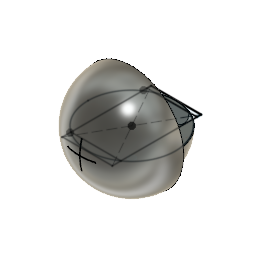
led-juggling-ball (Autodesk Fusion 360 design; units mm, degrees)
Autodesk Fusion 360 part; units mm, degrees
sketch "Sketch1" plane through (0, 0, 0) normal (0, 0, 1) x (1, 0, 0)
  circle A0 centre (0, 0) radius 37.5
  line L0 (-37.5, 0) -> (37.5, 0)
  circle A1 centre (0, 0) radius 33.25
  line L1 (-32.8653, 0.0244) -> (-33.25, 0)
  line L2 (0, 37.5) -> (0, 0)
  line L3 (0, 0) -> (0, -37.5)
  dimension "d1" = 75
  dimension "d2" = 66.5
  constraint coincident A0.centre A1.centre
  constraint coincident A0 L0.start
  constraint coincident A0 L0.end
  constraint horizontal L0
  constraint concentric A0 A1
  constraint coincident A1 L1.end
  constraint coincident L0 L1.end
  constraint coincident A0 L2.start
  constraint coincident A0 L3.end
  constraint perpendicular L0 L3
  measures "d1" diameter of A0
  measures "d2" diameter of A1
revolve "Revolve3" add sketch "Sketch1" angle 360 about axis through (0, 0, 0) along (0, -1, 0) contours A0 L0 A1 L3 picked at (-3.3563, -35.8433) makes body 1
revolve "Revolve2" add sketch "Sketch1" angle 360 about axis through (0, 37.5, 0) along (0, -1, 0) separate body contours A0 L0 A1 L2 picked at (-1.7789, 35.9561) makes body 2
sketch "Sketch2" plane through (0, 0, 0) normal (0, 1, 0) x (1, 0, 0)
  circle A0 centre (0, 0) radius 10
  dimension "d7" = 20
  constraint coincident A0.centre origin
  measures "d7" diameter of A0
extrude "Extrude1" cut sketch "Sketch2" against normal blind 60 bodies 1
sketch "Sketch3" plane through (0, 0, 0) normal (0, 0, 1) x (1, 0, 0)
  spline S0 degree 5 poles (0, -35) (0.4009, -35.0057) (1.2027, -35.0023) (2.4054, -34.9527) (4.0091, -34.8067) (6.012, -34.5127) (7.6108, -34.1894) (8.8068, -33.8887) (9.6025, -33.6595) (10, -33.5378) knots 0 0 0 0 0 0 0.2 0.4 0.6 0.8 1 1 1 1 1 1
  line L0 (-1.0163, -34.9855) -> (1.0163, -35.0145)
  line L1 (8.9918, -33.8467) -> (11.0081, -33.2288)
  line L2 (0, -35) -> (0, -31.5)
  line L3 (10, -33.5378) -> (10, -29.5378)
  line L4 (10, -29.5378) -> (11.8793, -28.8537)
  line L5 (11.8793, -28.8537) -> (11.8793, -28.4537)
  spline S1 degree 5 poles (11.8793, -28.4537) (11.8793, -28.4528) (11.7956, -28.4591) (11.4191, -28.4933) (10.6251, -28.5552) (9.9506, -28.5569) (9.9154, -28.5174) (9.5374, -28.7608) (8.5649, -29.3019) (6.9381, -30.0477) (4.8211, -30.8112) (2.912, -31.2735) (1.4544, -31.4588) (0.4845, -31.5) (0, -31.5) knots 0 0 0 0 0 0 0.1 0.2 0.3 0.4 0.5 0.6 0.7 0.8 0.9 1 1 1 1 1 1
  line L6 (10.242, -28.5357) -> (9.7191, -28.5641)
  line L7 (11.8793, -28.4607) -> (11.8793, -28.4468)
  line L8 (1.9201, -31.5) -> (-1.9201, -31.5)
  point P0 (9.9806, -28.5499)
  dimension "d10" = 4
  dimension "d11" = 110
  dimension "d12" = 2
  dimension "d13" = 0.4
  dimension "d61" = 3.5
  constraint midpoint S0.start L0
  constraint midpoint S0.end L1
  constraint vertical L3
  constraint vertical L5
  constraint midpoint P0 L6
  constraint midpoint L5.end L7
  constraint coincident L6 L7.end
  constraint midpoint L2.end L8
  constraint coincident L5 L7.start
  measures "d10" distance of S0.end L3.end
  measures "d11" angle of L3 L4
  measures "d12" distance of L3.end L4.end
  measures "d13" distance of L4.end L5.end
  measures "d61" distance of S0.start L2.end
sketch "Sketch4" plane through (0, 0, 0) normal (0, 0, 1) x (1, 0, 0)
  line L0 (10, -33.5) -> (10, -30.5)
  spline S0 degree 5 poles (0, -35) (0.3549, -35) (1.0653, -34.9917) (2.133, -34.9543) (3.5701, -34.8539) (5.4548, -34.6187) (7.113, -34.2978) (8.4939, -33.948) (9.486, -33.6587) (10, -33.5) knots 0 0 0 0 0 0 0.2 0.4 0.6 0.8 1 1 1 1 1 1
  line L1 (8.6967, -33.9024) -> (11.3033, -33.0976)
  line L2 (-0.9, -35) -> (0.9, -35)
  line L3 (10, -30.5) -> (8, -30.5)
  line L4 (0, -35) -> (0, -33)
  spline S1 degree 5 poles (0, -33) (0.7014, -32.9425) (1.9674, -32.8352) (3.4564, -32.6972) (4.7558, -32.5362) (5.7676, -32.2435) (6.495, -31.7925) (7.1733, -31.2433) (7.7103, -30.7663) (8, -30.5) knots 0 0 0 0 0 0 0.2 0.4 0.6 0.8 1 1 1 1 1 1
  line L5 (-1.7671, -33.1448) -> (1.7671, -32.8552)
  line L6 (7.2949, -31.1481) -> (8.7051, -29.8519)
  dimension "d15" = 3
  dimension "d22" = 2
  constraint vertical L0
  constraint midpoint L0.start L1
  constraint midpoint S0.start L2
  constraint perpendicular L0 L3
  constraint vertical L4
  constraint midpoint L4.end L5
  constraint midpoint L3.end L6
  measures "d15" distance of L0.start L0.end
  measures "d22" distance of L0.end L3.end
sketch "Sketch6" plane through (0, 0, 0) normal (0, 1, 0) x (1, 0, 0)
  line L0 (-32, 0) -> (0, 0)
  line L1 (0, 0) -> (0, 32)
  circle A0 centre (0, 0) radius 32
  dimension "d103" = 64
  constraint coincident L0.end L1.start
  constraint horizontal L0
  constraint perpendicular L0 L1
  constraint coincident L1.end A0
  measures "d103" diameter of A0
revolve "Revolve6" add sketch "Sketch6" angle 360 about axis through (0, 0, 0) along (0, 0, -1) separate body contours L0 L1 A0 picked at (-21.2248, 1.518) makes body 3
sketch "Sketch7" plane through (0, 0, 0) normal (0, 0, 1) x (-1, 0, 0)
  circle A0 centre (0, 0) radius 32
  line L0 (18, 32) -> (-18, 32)
  line L1 (-18, 32) -> (-18, -32)
  line L2 (-18, -32) -> (18, -32)
  line L3 (18, -32) -> (18, 32)
  line L4 (18, 32) -> (-18, -32) construction
  line L5 (-18, 32) -> (18, -32) construction
  line L6 (18, -32) -> (-18, -32)
  line L7 (-18, -32) -> (-18, -29)
  line L8 (-18, -29) -> (18, -29)
  line L9 (18, -29) -> (18, -32)
  circle A1 centre (0, 0) radius 31.5
  line L10 (18, 25.8505) -> (-18, 25.8505)
  point P0 (18, -26.4575)
  point P1 (18, 26.4575)
  dimension "d24" = 36
  dimension "d25" = 64
  dimension "d26" = 3
  dimension "d29" = 63
  constraint horizontal L0
  constraint perpendicular L0 L1
  constraint parallel L0 L2
  constraint parallel L1 L3
  constraint coincident L4 A0.centre
  constraint coincident L5 A0.centre
  constraint coincident A0.centre A1.centre
  constraint coincident L3 P0
  constraint coincident A0 P0
  constraint coincident L3 P1
  constraint coincident A0 P1
  constraint horizontal L6
  constraint vertical L7
  constraint horizontal L8
  constraint vertical L9
  constraint coincident L3 L10.start
  constraint coincident A1 L10.start
  constraint coincident L1 L10.end
  constraint coincident A1 L10.end
  measures "d24" distance of L1.end L2.end
  measures "d25" distance of L0.end L1.end
  measures "d26" distance of L2.end L8.end
  measures "d29" diameter of A1
extrude "Extrude4" cut sketch "Sketch7" against normal blind 12.5 contours L1 L3 L8 A1 L10 bodies 3
sketch "Sketch8" plane through (0, 0, -12.5) normal (0, 0, 1) x (-1, 0, 0)
  arc A0 (18, 23.3184) -> (14.1244, 25.8505) centre (0, 0) ccw
  line L0 (-18, 23.3184) -> (-18, -23.3184)
  arc A1 (-18, -23.3184) -> (-5.172, -29) centre (0, 0) ccw
  line L1 (-5.172, -29) -> (5.172, -29)
  arc A2 (5.172, -29) -> (18, -23.3184) centre (0, 0) ccw
  line L2 (18, -23.3184) -> (18, 23.3184)
  circle A3 centre (0, 0) radius 2.5
  line L3 (14.1244, 25.8505) -> (-14.1244, 25.8505)
  arc A4 (-14.1244, 25.8505) -> (-18, 23.3184) centre (0, 0) ccw
  dimension "d32" = 5
  constraint concentric A0 A3
  measures "d32" diameter of A3
extrude "Extrude5" cut sketch "Sketch8" against normal blind 1 contours A3 bodies 3
sketch "Sketch9" plane through (0, 0, 0) normal (1, 0, 0) x (0, 1, 0)
  line L0 (0, 0) -> (32, 0)
  line L1 (0, 0) -> (0, -32)
  circle A0 centre (0, 0) radius 32
  circle A1 centre (0, 0) radius 31.5
  dimension "d35" = 63
  constraint coincident L0.start L1.start
  constraint horizontal L0
  constraint perpendicular L0 L1
  constraint coincident L1.end A0
  measures "d35" diameter of A1
revolve "Revolve7" add sketch "Sketch9" angle 360 about axis through (0, 0, 0) along (0, 0, -1) contours L0 L1 A0 A1 picked at (31.6179, -3.0123) bodies 3
sketch "Sketch10" plane through (0, -25.8505, 0) normal (0, 1, 0) x (-1, 0, 0)
  arc A0 (-18, 0) -> (-12.9518, -12.5) centre (0, 0) ccw
  line L0 (-12.9518, -12.5) -> (12.9518, -12.5)
  arc A1 (12.9518, -12.5) -> (18, 0) centre (0, 0) ccw
  line L1 (18, 0) -> (-18, 0)
  circle A2 centre (0, 0) radius 12.5
  constraint concentric A0 A2
  constraint tangent L0 A2
extrude "Extrude6" cut sketch "Sketch10" against normal blind 10 from surface at -0.5 contours L1 A2 picked at (-3.149, -3.9145) bodies 3
sketch "Sketch11" plane through (0, 0, -12.5) normal (0, 0, 1) x (-1, 0, 0)
  circle A0 centre (0, 0) radius 2.5
  line L0 (18, -22.6274) -> (18, 22.6274)
  arc A1 (18, 22.6274) -> (12.9518, 25.8505) centre (0, 0) ccw
  line L1 (12.9518, 25.8505) -> (-12.9518, 25.8505)
  arc A2 (-12.9518, 25.8505) -> (-18, 22.6274) centre (0, 0) ccw
  line L2 (-18, 22.6274) -> (-18, -22.6274)
  arc A3 (-18, -22.6274) -> (18, -22.6274) centre (0, 0) ccw
  line L3 (16, -23) -> (-10, -23)
  line L4 (-10, -23) -> (-10, -13)
  line L5 (-10, -13) -> (16, -13)
  line L6 (16, -13) -> (16, -23)
  dimension "d40" = 10
  dimension "d43" = 26
  constraint horizontal L3
  constraint vertical L4
  constraint horizontal L5
  constraint vertical L6
  measures "d40" distance of L3.start L5.end
  measures "d43" distance of L3.start L3.end
extrude "Extrude7" add sketch "Sketch11" along normal blind 2 separate body contours L3 L4 L5 L6 makes body 4
sketch "Sketch12" plane through (0, 0, -12.5) normal (0, 0, 1) x (-1, 0, 0)
  circle A0 centre (0, 0) radius 2.5
  line L0 (18, -22.6274) -> (18, 22.6274)
  arc A1 (18, 22.6274) -> (12.9518, 25.8505) centre (0, 0) ccw
  line L1 (12.9518, 25.8505) -> (-12.9518, 25.8505)
  arc A2 (-12.9518, 25.8505) -> (-18, 22.6274) centre (0, 0) ccw
  line L2 (-18, 22.6274) -> (-18, -22.6274)
  arc A3 (-18, -22.6274) -> (18, -22.6274) centre (0, 0) ccw
  line L3 (-10, 20) -> (10, 20)
  line L4 (10, 20) -> (10, 10)
  line L5 (10, 10) -> (-10, 10)
  line L6 (-10, 10) -> (-10, 20)
  dimension "d44" = 20
  dimension "d45" = 10
  constraint horizontal L3
  constraint vertical L4
  constraint horizontal L5
  constraint vertical L6
  measures "d44" distance of L3.start L3.end
  measures "d45" distance of L3.start L5.end
extrude "Extrude8" add sketch "Sketch12" along normal blind 2 separate body contours L3 L4 L5 L6 makes body 5
sketch "Sketch13" plane through (0, 0, -12.5) normal (0, 0, 1) x (-1, 0, 0)
  circle A0 centre (0, 0) radius 2.5
  line L0 (18, -22.6274) -> (18, 22.6274)
  arc A1 (18, 22.6274) -> (12.9518, 25.8505) centre (0, 0) ccw
  line L1 (12.9518, 25.8505) -> (-12.9518, 25.8505)
  arc A2 (-12.9518, 25.8505) -> (-18, 22.6274) centre (0, 0) ccw
  line L2 (-18, 22.6274) -> (-18, -22.6274)
  arc A3 (-18, -22.6274) -> (18, -22.6274) centre (0, 0) ccw
  line L3 (6, 9) -> (-6, 9)
  line L4 (-6, 9) -> (-6, 12)
  line L5 (-6, 12) -> (6, 12)
  line L6 (6, 12) -> (6, 9)
  dimension "d48" = 12
  dimension "d49" = 3
  constraint horizontal L3
  constraint vertical L4
  constraint horizontal L5
  constraint vertical L6
  measures "d48" distance of L3.start L3.end
  measures "d49" distance of L3.start L5.end
extrude "Extrude9" add sketch "Sketch13" along normal blind 3.8 separate body contours L3 L4 L5 L6 makes body 6
sketch "Sketch14" plane through (0, 0, -12.5) normal (0, 0, 1) x (-1, 0, 0)
  circle A0 centre (0, 0) radius 2.5
  line L0 (18, -22.6274) -> (18, 22.6274)
  arc A1 (18, 22.6274) -> (12.9518, 25.8505) centre (0, 0) ccw
  line L1 (12.9518, 25.8505) -> (-12.9518, 25.8505)
  arc A2 (-12.9518, 25.8505) -> (-18, 22.6274) centre (0, 0) ccw
  line L2 (-18, 22.6274) -> (-18, -22.6274)
  arc A3 (-18, -22.6274) -> (18, -22.6274) centre (0, 0) ccw
  line L3 (6, 9) -> (-2, 9)
  line L4 (-2, 9) -> (-2, 17)
  line L5 (-2, 17) -> (6, 17)
  line L6 (6, 17) -> (6, 9)
  dimension "d52" = 8
  dimension "d53" = 8
  constraint horizontal L3
  constraint vertical L4
  constraint horizontal L5
  constraint vertical L6
  measures "d52" distance of L3.start L3.end
  measures "d53" distance of L3.start L5.end
extrude "Extrude10" add sketch "Sketch14" along normal blind 2 separate body contours L3 L4 L5 L6 makes body 7
sketch "Sketch15" plane through (0, 0, 0) normal (0, 1, 0) x (1, 0, 0)
  line L0 (-5, 1) -> (5, 1)
  line L1 (5, 1) -> (5, -1)
  line L2 (5, -1) -> (-5, -1)
  line L3 (-5, -1) -> (-5, 1)
  line L4 (-5, 1) -> (5, -1) construction
  line L5 (5, 1) -> (-5, -1) construction
  dimension "d56" = 10
  constraint horizontal L0
  constraint perpendicular L0 L1
  constraint parallel L0 L2
  constraint parallel L1 L3
  constraint coincident L4 origin
  constraint coincident L5 origin
  measures "d56" distance of L1.end L2.end
sketch "Sketch18" plane through (0, 0, 0) normal (0, 0, 1) x (1, 0, 0)
  line L0 (34.6845, 0.0935) -> (36.0845, 0.0935)
  spline S0 degree 5 poles (34.6845, 0.0935) (34.7506, -0.1078) (34.8946, -0.4756) (35.1459, -0.9233) (35.543, -1.3466) (36.1191, -1.7241) (36.6345, -2.012) (37.0533, -2.2677) (37.348, -2.4629) (37.4992, -2.5667) knots 0 0 0 0 0 0 0.2 0.4 0.6 0.8 1 1 1 1 1 1
  line L1 (34.487, 0.6947) -> (34.882, -0.5077)
  line L2 (37.0231, -2.2399) -> (37.9752, -2.8934)
  spline S1 degree 5 poles (36.0845, 0.0935) (36.1093, 0.0042) (36.162, -0.1638) (36.2504, -0.3842) (36.3899, -0.6269) (36.6278, -0.896) (36.9073, -1.1275) (37.1942, -1.3322) (37.4255, -1.486) (37.5511, -1.5672) knots 0 0 0 0 0 0 0.2 0.4 0.6 0.8 1 1 1 1 1 1
  line L3 (36.0269, 0.301) -> (36.1422, -0.114)
  line L4 (37.25, -1.3725) -> (37.8522, -1.762)
  line L5 (37.4992, -2.5667) -> (37.5511, -1.5672)
  spline S2 degree 5 poles (36.0845, 0.0935) (36.1093, 0.1828) (36.162, 0.3508) (36.2504, 0.5713) (36.3899, 0.8139) (36.6278, 1.083) (36.9073, 1.3145) (37.1942, 1.5192) (37.4255, 1.673) (37.5511, 1.7543) knots 0 0 0 0 0 0 0.2 0.4 0.6 0.8 1 1 1 1 1 1
  line L6 (36.0269, -0.114) -> (36.1422, 0.301)
  line L7 (37.25, 1.5595) -> (37.8522, 1.949)
  line L8 (37.4992, 2.7537) -> (37.5511, 1.7543)
  spline S3 degree 5 poles (34.6845, 0.0935) (34.7506, 0.2948) (34.8946, 0.6626) (35.1459, 1.1103) (35.543, 1.5336) (36.1191, 1.9111) (36.6345, 2.199) (37.0533, 2.4547) (37.348, 2.6499) (37.4992, 2.7537) knots 0 0 0 0 0 0 0.2 0.4 0.6 0.8 1 1 1 1 1 1
  line L9 (34.487, -0.5077) -> (34.882, 0.6947)
  line L10 (37.0231, 2.427) -> (37.9752, 3.0805)
  dimension "d75" = 1.4
  constraint horizontal L0
  constraint symmetric L0 S0.start S3.start
  constraint symmetric L0 S0.end L8.start
  constraint symmetric L0 L1.start L9.start
  constraint symmetric L0 L1.end L9.end
  constraint symmetric L0 L2.start L10.start
  constraint symmetric L0 L2.end L10.end
  constraint symmetric L0 S1.start S2.start
  constraint symmetric L0 S1.end S2.end
  constraint symmetric L0 L3.start L6.start
  constraint symmetric L0 L3.end L6.end
  constraint symmetric L0 L4.start L7.start
  constraint symmetric L0 L4.end L7.end
  constraint midpoint S0.end L2
  measures "d75" distance of L0.start L0.end
extrude "Extrude14" [suppressed]
pattern_circular "C-Pattern1" [suppressed]
extrude "Extrude16" cut 1 faces at (-0.7914, 0.9038, -13.5) along direction (0, 0, -1) blind 6.5 on bodies 3 bodies 3
sketch "Sketch20" plane through (0, 0, -20) normal (0, 0, 1) x (-1, 0, 0)
  circle A0 centre (0, 0) radius 2.5
fillet "Fillet1" radius 1.5 1 edges at (2.3308, -0.904, -20) on bodies 3
sketch "Sketch21" plane through (0, -26.3505, 0) normal (0, -1, 0) x (1, 0, 0)
  line L0 (12.5, 0) -> (-12.5, 0)
  arc A0 (-12.5, 0) -> (12.5, 0) centre (0, 0) ccw
  line L1 (4.5, -7) -> (-4.5, -7)
  line L2 (-4.5, -7) -> (-4.5, 7)
  line L3 (-4.5, 7) -> (4.5, 7)
  line L4 (4.5, 7) -> (4.5, -7)
  line L5 (4.5, -7) -> (-4.5, 7) construction
  line L6 (-4.5, -7) -> (4.5, 7) construction
  dimension "d82" = 9
  dimension "d83" = 14
  constraint horizontal L1
  constraint perpendicular L1 L2
  constraint parallel L1 L3
  constraint parallel L2 L4
  constraint coincident L5 A0.centre
  constraint coincident L6 A0.centre
  constraint coincident A0.centre origin
  measures "d82" distance of L2.end L3.end
  measures "d83" distance of L1.end L2.end
extrude "Extrude17" cut sketch "Sketch21" against normal blind 6.5 contours L0 L1 L2 L4 bodies 3
fillet "Fillet2" radius 1 2 edges at (-4.5, -26.1005, -7) (4.5, -26.1005, -7) on bodies 3
sketch "Sketch24" plane through (0, 0, 0) normal (0, 0, 1) x (1, 0, 0)
  circle A0 centre (0, 0) radius 37.5
  circle A1 centre (0, 0) radius 36.5
  line L0 (0, 0) -> (0, -37.5)
  line L1 (0, 0) -> (-22.4943, -30.0043)
  dimension "d94" = 75
  dimension "d95" = 73
  constraint coincident A0.centre A1.centre
  constraint concentric A0 A1
  constraint coincident A0 L0.end
  constraint vertical L0
  constraint coincident A0 L1.end
  measures "d94" diameter of A0
  measures "d95" diameter of A1
revolve "Revolve8" add sketch "Sketch24" angle 360 about axis through (0, 0, 0) along (0, -1, 0) contours A0 A1 L0 L1 picked at (-3.1649, -36.9628) bodies 1
sketch "Sketch25" plane through (0, 0, 0) normal (0, 1, 0) x (1, 0, 0)
  line L0 (0.25, 10) -> (-0.25, 10)
  line L1 (-0.25, 10) -> (-0.25, -10)
  line L2 (-0.25, -10) -> (0.25, -10)
  line L3 (0.25, -10) -> (0.25, 10)
  line L4 (0.25, 10) -> (-0.25, -10) construction
  line L5 (-0.25, 10) -> (0.25, -10) construction
  line L6 (-10, 0.25) -> (10, 0.25)
  line L7 (10, 0.25) -> (10, -0.25)
  line L8 (10, -0.25) -> (-10, -0.25)
  line L9 (-10, -0.25) -> (-10, 0.25)
  line L10 (-10, 0.25) -> (10, -0.25) construction
  line L11 (10, 0.25) -> (-10, -0.25) construction
  dimension "d97" = 0.5
  dimension "d98" = 20
  dimension "d99" = 20
  dimension "d100" = 0.5
  constraint horizontal L0
  constraint perpendicular L0 L1
  constraint parallel L0 L2
  constraint parallel L1 L3
  constraint coincident L4 origin
  constraint coincident L5 origin
  constraint horizontal L6
  constraint perpendicular L6 L7
  constraint parallel L6 L8
  constraint parallel L7 L9
  constraint coincident L10 origin
  constraint coincident L11 origin
  measures "d97" distance of L1.end L2.end
  measures "d98" distance of L0.end L1.end
  measures "d99" distance of L7.end L8.end
  measures "d100" distance of L6.end L7.end
extrude "Extrude21" cut sketch "Sketch25" along normal mid plane 200 bodies 1
hidden bodies 2 4 5 6 7
equation "d62 = -2147483647.n mm"
named bodies: "outer-back", "outer-front", "inner-1", "battery-bottom-spacer", "esp-bottom-spacer", "tp-spacer", "accel-spacer"
